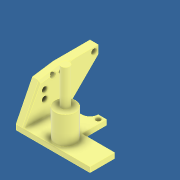
# Autodesk Inventor part: HolderShaft
Saved by Autodesk Inventor 2020 (Build 240168000, 168)
## iProperties
Created: 2019-12-14
Part Number: HolderShaft
Material: ABS Plastic
Document SubType Name: Modeling
Designer: Jack
Density: 1.06 g/cm^3
Appearance: Smooth - White
Author: Jack
Autodesk Inventor part; units mm, degrees
ref_plane "YZ Plane" through (0, 0, 0) normal (1, 0, 0) x (0, 1, 0)
ref_plane "XZ Plane" through (0, 0, 0) normal (0, 1, 0) x (-1, 0, 0)
ref_plane "Work Plane1" through (-8.8205, 35.5, -8.8205) normal (0, 1, 0) x (0.309017, 0, 0.9510565)
sketch "Sketch1" plane through (0, 0, 0) normal (0, 1, 0) x (-1, 0, 0)
  circle A0 centre (0, 0) radius 4
  dimension "d0" = 8
  constraints: 1 centre point, 1 coincident
  measures "d0" diameter of A0
extrude "Extrusion1" add sketch "Sketch1" along normal up to surface (35.5 mm away)
sketch "Sketch5" plane through (0, 0, 0) normal (0, -1, 0) x (1, 0, 0)
  circle A0 centre (0, 0) radius 10
  dimension "d17" = 20
  constraints: 1 centre point, 1 coincident
  measures "d17" diameter of A0
extrude "Extrusion3" add sketch "Sketch5" along normal blind 27
sketch "Sketch17" plane through (0, -27, 0) normal (0, -1, 0) x (1, 0, 0)
  line L0 (36, 12) -> (-36, 12)
  line L1 (-36, 12) -> (-36, -12)
  line L2 (-36, -12) -> (36, -12)
  line L3 (36, -12) -> (36, 12)
  line L4 (36, 12) -> (-36, -12) construction
  line L5 (-36, 12) -> (36, -12) construction
  point P0 (0, 0)
  point P1 (0, 0)
  point P2 (0, 0)
  dimension "d86" = 72
  dimension "d87" = 24
  constraints: 12 end point, 3 midpoint, 2 parallel, 1 coincident, 1 horizontal, 1 perpendicular
  measures "d86" distance of L1.end L2.end
  measures "d87" distance of L0.end L1.end
extrude "Extrusion9" add sketch "Sketch17" along normal blind 5
pattern_circular "Circular Pattern1" count 4 over 360 about axis through (0, -10, 0) along (0, 1, 0)
sketch "Sketch19" plane through (0, -27, 0) normal (0, 1, 0) x (1, 0, 0)
  line L0 (-36, -12) -> (-36, 12) projected
  line L1 (-36, 12) -> (-28, 12)
  line L2 (-28, 12) -> (-28, 4)
  line L3 (-28, 4) -> (-36, 4)
  line L4 (-36, 4) -> (-36, 12)
  point P0 (0, 0)
  point P1 (-36, 4)
  dimension "d103" = 8
  dimension "d104" = 8
  constraints: 8 end point, 2 parallel, 1 horizontal, 1 perpendicular
  measures "d103" distance of L2.end L3.end
  measures "d104" distance of L1.end L2.end
extrude "Extrusion11" add sketch "Sketch19" along normal blind 35
sketch "Sketch20" plane through (-12, -32, -12) normal (0, 0, -1) x (-1, 0, 0)
  line L0 (16, 5) -> (16, 40) projected
  line L1 (16, 40) -> (24, 40)
  line L2 (24, 40) -> (24, 0)
  line L3 (24, 0) -> (16, 0)
  line L4 (16, 0) -> (16, 40)
  point P0 (-12, 32)
  dimension "d107" = 8
  dimension "d108" = 40
  constraints: 8 end point, 2 parallel, 1 horizontal, 1 perpendicular
  measures "d107" distance of L2.end L3.end
  measures "d108" distance of L1.end L2.end
extrude "Extrusion12" add sketch "Sketch20" along normal blind 48
chamfer "Chamfer4" distance 32 angle 45 1 edges at (-32, -32, -60)
chamfer "Chamfer5" distance 20 distance2 3 1 edges at (-32, 8, -4) measured on face at (-32, 8, -4.5)
chamfer "Chamfer6" distance 2 angle 45 1 edges at (-28, 6.5, -14)
sketch "Sketch21" plane through (-36, -32, 12) normal (-1, 0, 0) x (0, 0, 1)
  line L0 (-16, 5) -> (-16, 37) projected
  line L1 (0, 5) -> (-16, 5) projected
  line L2 (-16, 37) -> (0, 5)
  point P0 (-12, 32)
  constraints: 2 end point
extrude "Extrusion13" add sketch "Sketch21" against normal blind 6
sketch "Sketch23" plane through (-28, -27, -4) normal (1, 0, 0) x (0, 0, -1)
  line L0 (0, 0) -> (0, 29.9776) projected
  line L1 (0, 0) -> (-16, 0) projected
  line L2 (0, 29.9776) -> (-16, 0)
  point P0 (-4, 27)
  constraints: 2 end point
loft "Loft1" add profiles "Sketch23" section 2 edges at (-30, -11, 4) (-30, -27, 4) (-30, -11, -4)
sketch "Sketch24" plane through (-36, 0, -60) normal (-1, 0, 0) x (0, 0, 1)
  circle A0 centre (52, -4.0333) radius 2.4
  circle A1 centre (52, -12.0333) radius 2.4
  circle A2 centre (44, 3.9667) radius 2.4
  circle A3 centre (36, 3.9667) radius 2.4
  circle A4 centre (4, 3.9667) radius 2.4
  line L0 (72, -27) -> (72, -32) projected
  point P0 (60, 0)
  dimension "d126" = 4.8
  dimension "d127" = 4.8
  dimension "d128" = 4.8
  dimension "d129" = 4.8
  dimension "d130" = 4.8
  dimension "d131" = 8
  dimension "d132" = 8
  dimension "d133" = 8
  dimension "d134" = 8
  dimension "d135" = 32
  dimension "d136" = 20
  constraints: 5 centre point, 2 horizontal alignment, 1 vertical alignment
  measures "d126" diameter of A0
  measures "d127" diameter of A1
  measures "d128" diameter of A2
  measures "d129" diameter of A3
  measures "d130" diameter of A4
  measures "d131" distance of A0.centre A1.centre
  measures "d132" horizontal distance of A0.centre A2.centre
  measures "d133" distance of A2.centre A3.centre
  measures "d134" horizontal distance of A0.centre A2.centre
  measures "d135" distance of A4.centre A3.centre
  measures "d136" distance from line of L0 A1.centre
extrude "Extrusion14" cut sketch "Sketch24" against normal blind 16
fillet "Fillet1" radius 0.7 10 edges at (-36, 3.9667, -58.4) (-28, 3.9667, -58.4) (-36, 3.9667, -26.4) (-36, 3.9667, -18.4) (-28, 1.6382, -16.5817) (-28, 4.1965, -13.611) (-36, -4.0333, -10.4) (-28, -4.0333, -10.4) (-36, -12.0333, -10.4) (-28, -12.0333, -10.4)
sketch "Sketch25" plane through (0, -32, 0) normal (0, -1, 0) x (1, 0, 0)
  circle A0 centre (0, -32) radius 2.4
  point P0 (0, 0)
  dimension "d140" = 4.8
  dimension "d141" = 32
  constraints: 1 centre point, 1 vertical alignment
  measures "d140" diameter of A0
  measures "d141" distance of A0.centre point (0, 0)
extrude "Extrusion15" cut sketch "Sketch25" against normal blind 16
sketch "Sketch27" plane through (12, -32, 12) normal (1, 0, 0) x (0, 0, -1)
  line L0 (0, 5) -> (0, 0) projected
  line L1 (0, 5) -> (-24, 5) projected
  line L2 (-24, 5) -> (-24, 0) projected
  line L3 (0, 0) -> (-24, 0) projected
  point P0 (12, 32)
extrude "Extrusion16" cut sketch "Sketch27" against normal blind 32
sketch "Sketch28" plane through (12, -32, -12) normal (1, 0, 0) x (0, 0, -1)
  line L0 (0, 0) -> (0, 5) projected
  line L1 (24, 0) -> (0, 0) projected
  line L2 (24, 5) -> (24, 0) projected
  line L3 (24, 5) -> (0, 5) projected
  point P0 (-12, 32)
extrude "Extrusion17" cut sketch "Sketch28" against normal blind 8
sketch "Sketch31" plane through (-12, -32, -12) normal (-1, 0, 0) x (0, 0, 1)
  line L0 (0, 0) -> (-24, 0) projected
  line L1 (0, 5) -> (0, 0) projected
  line L2 (0, 5) -> (-24, 5) projected
  line L3 (-24, 5) -> (-24, 0) projected
  point P0 (12, 32)
extrude "Extrusion19" cut sketch "Sketch31" against normal blind 8
sketch "Sketch33" plane through (0, -32, 0) normal (0, -1, 0) x (1, 0, 0)
  line L0 (-4, -12) -> (-4, -36) projected
  line L1 (-28, -12) -> (-28, -28) projected
  line L2 (-28, -12) -> (-4, -12) projected
  line L3 (-28, -60) -> (-28, -28) projected
  line L4 (-28, -28) -> (-12, -28)
  arc A0 (-4, -36) -> (-12, -28) centre (-12, -36) ccw
  point P0 (0, 0)
  dimension "d156" = 16
  constraints: 2 end point, 2 point on circle, 1 centre point, 1 horizontal, 1 tangent
  measures "d156" distance of L1.end L4.end
extrude "Extrusion20" add sketch "Sketch33" against normal blind 5
body "Solid1"
